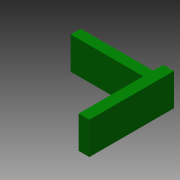
# Autodesk Inventor part: MudGuard
Saved by Autodesk Inventor 2014 SP1 (Build 180222100, 222)
## iProperties
Created: 2017-01-19
Part Number: MudGuard
Material: Generic
Document SubType Name: Modeling
Designer: danielsikar
Density: 1 g/cm^3
Appearance: Dark Green
Author: danielsikar
Autodesk Inventor part; units mm, degrees
ref_plane "YZ Plane" through (0, 0, 0) normal (1, 0, 0) x (0, 1, 0)
ref_plane "XZ Plane" through (0, 0, 0) normal (0, 1, 0) x (-1, 0, 0)
ref_plane "XY Plane" through (0, 0, 0) normal (0, 0, 1) x (1, 0, 0)
sketch "Sketch3" plane through (0, 0, 0) normal (0, 0, 1) x (1, 0, 0)
  line L0 (0, 0) -> (-20, 0) construction
  line L1 (-20, 0) -> (-20, 28) construction
  line L2 (-20, 28) -> (0, 28) construction
  line L3 (0, 28) -> (0, 0) construction
  line L4 (0, 0) -> (-5, 0)
  line L5 (-5, 39.2612) -> (0, 39.2612)
  line L6 (0, 39.2612) -> (0, 0)
  line L7 (-7, 39.2612) -> (-7, 17.5337) construction
  circle A0 centre (-7, 28) radius 2
  line L8 (-38.6834, 30) -> (-38.6834, 34.6231)
  line L9 (-38.6834, 34.6231) -> (2.4889, 34.6231)
  line L10 (2.4889, 34.6231) -> (2.4889, 30)
  line L11 (2.4889, 30) -> (-0.2918, 30)
  line L12 (-5, 30) -> (-38.6834, 30)
  line L13 (-5, 0) -> (-5, 30)
  line L14 (-5, 34.6231) -> (-5, 39.2612)
  arc A1 (0, 28) -> (-9.2658, 34.6231) centre (-7, 28) ccw
  arc A2 (-13.7082, 30) -> (-5, 21.2918) centre (-7, 28) ccw
  dimension "d20" = 20
  dimension "d21" = 28
  dimension "d22" = 5
  dimension "d23" = 7
  constraints: 30 end point, 9 parallel, 7 point on line, 5 perpendicular, 5 point on circle, 4 horizontal, 3 centre point, 1 coincident, 1 tangent
  measures "d20" distance of L2.end L1.end
  measures "d21" distance of L0.end L1.end
  measures "d22" distance of L5.start L5.end
  measures "d23" distance between parallel lines of L7 L6
extrude "Extrusion2" add sketch "Sketch3" along normal blind 15 contours L4 L13 L12 L8 L9 A1 L6 | A1 L11 L6 | L11 A1 L9 L6 | L9 A1 L14 L5 L6 | L9 L14 A1 picked at (-4.8521, 34.6329)
body "Solid2"
